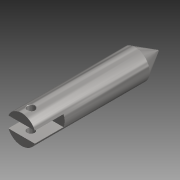
# Autodesk Inventor part: solenoid pin
Saved by Autodesk Inventor 2014 (Build 180170000, 170)
## iProperties
Created: 2013-07-22
Part Number: solenoid pin
Material: Generic
Document SubType Name: Modeling
Designer: Saville
Mass: 5.89525 g
Surface Area: 25.6095 cm^2
Volume: 5.89525 cm^3
Density: 1 g/cm^3
Appearance: Default
Author: Saville
Autodesk Inventor part; units mm, degrees
ref_plane "YZ Plane" through (0, 0, 0) normal (1, 0, 0) x (0, 1, 0)
ref_plane "XZ Plane" through (0, 0, 0) normal (0, 1, 0) x (-1, 0, 0)
ref_plane "XY Plane" through (0, 0, 0) normal (0, 0, 1) x (1, 0, 0)
sketch "Sketch1" plane through (0, 0, 0) normal (0, 0, 1) x (1, 0, 0)
  circle A0 centre (0, 0) radius 6.3309
  dimension "d0" = 12.6619
  constraints: 1 centre point, 1 coincident
  measures "d0" diameter of A0
extrude "Extrusion1" add sketch "Sketch1" against normal blind 60.0964
sketch "Sketch2" plane through (0, 0, 0) normal (0, 1, 0) x (-1, 0, 0)
  line L0 (-6.3309, -60.0964) -> (-6.3309, 0) projected
  line L1 (-6.3309, 0) -> (6.3309, 0) projected
  line L2 (6.3309, 0) -> (6.3309, -60.0964) projected
  line L3 (6.3309, -60.0964) -> (-6.3309, -60.0964) projected
  line L4 (6.3309, -12.573) -> (-6.3309, -12.573)
  point P0 (0, 0)
  dimension "d3" = 12.573
  constraints: 2 end point, 2 point on line, 1 parallel
  measures "d3" distance between parallel lines of L4 L1
extrude "Extrusion2" cut sketch "Sketch2" along normal mid plane 4.9403 contours L0 L1 L2 L4
sketch "Sketch3" plane through (0, 2.4702, 0) normal (0, -1, 0) x (1, 0, 0)
  line L0 (-5.8292, 0) -> (5.8292, 0) construction
  line L1 (5.8292, 0) -> (5.8292, -12.573) construction
  line L2 (-5.8292, -12.573) -> (5.8292, -12.573) construction
  line L3 (-5.8292, -60.0964) -> (-5.8292, -12.573) construction
  line L4 (5.8292, -60.0964) -> (-5.8292, -60.0964) construction
  line L5 (5.8292, -12.573) -> (5.8292, -60.0964) construction
  line L6 (-5.8292, -12.573) -> (-5.8292, 0) construction
  line L7 (0, 0) -> (0, -12.573) construction
  circle A0 centre (0, -4.064) radius 1.651
  dimension "d6" = 3.302
  dimension "d7" = 4.064
  constraints: 2 end point, 1 centre point, 1 midpoint, 1 point on line
  measures "d6" diameter of A0
  measures "d7" distance from line of L0 A0.centre
extrude "Extrusion3" cut sketch "Sketch3" along normal through all both and the other way through all
sketch "Sketch4" plane through (0, 0, 0) normal (0, 1, 0) x (-1, 0, 0)
  line L0 (-6.3309, -12.573) -> (6.3309, -12.573) projected
  line L1 (6.3309, -12.573) -> (6.3309, -60.0964) projected
  line L2 (6.3309, -60.0964) -> (-6.3309, -60.0964) projected
  line L3 (-6.3309, -60.0964) -> (-6.3309, -12.573) projected
  line L4 (0, -60.0964) -> (0, -48.5629) construction
  line L5 (6.3309, -49.911) -> (0.3196, -59.9156)
  arc A0 (0, -60.0964) -> (0.3196, -59.9156) centre (0, -59.7236) ccw
  line L6 (0, -72.1662) -> (0, 12.0277) projected
  point P0 (0, 0)
  dimension "d10" = 10.1854
  dimension "d11" = 31
  constraints: 4 end point, 2 point on circle, 2 point on line, 2 tangent, 1 centre point, 1 midpoint, 1 parallel
  measures "d10" distance of L1.end L5.start
  measures "d11" angle of L1 L5
revolve "Revolution1" cut sketch "Sketch4" angle 360 about axis through (0, 0, -10) along (0, 0, 1) contours A0 L5 L1 L2
fillet "Fillet1" radius 0.0762 2 edges at (0, -6.3309, -49.911) (0, 6.3309, -49.911)
fillet "Fillet2" radius 0.127 2 edges at (0, -6.3309, 0) (0, 6.3309, 0)
chamfer "Chamfer1" distance 0.127 angle 45 2 edges at (-1.651, -6.1119, -4.0553) (-1.651, 6.1119, -4.0553)
body "Solid1"
